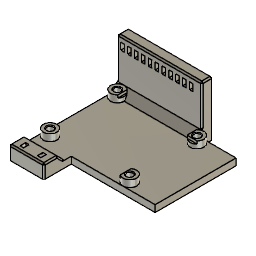
Pi Mount v3 (Autodesk Fusion 360 design; units mm, degrees)
Autodesk Fusion 360 part; units mm, degrees
note: some values were not read from the file. Set by a fixed rule: which sketch regions a step uses.
sketch "Sketch1" plane through (0, 0, 0) normal (0, 0, 1) x (1, 0, 0)
  line L0 (0, 0) -> (85, 0) construction
  line L1 (85, 0) -> (85, 56) construction
  line L2 (85, 56) -> (0, 56) construction
  line L3 (0, 56) -> (0, 0) construction
  line L4 (61.5, 3.5) -> (3.5, 3.5) construction
  line L5 (3.5, 3.5) -> (3.5, 52.5) construction
  line L6 (3.5, 52.5) -> (61.5, 52.5) construction
  line L7 (61.5, 52.5) -> (61.5, 3.5) construction
  line L8 (61.5, 3.5) -> (3.5, 52.5) construction
  line L9 (3.5, 3.5) -> (61.5, 52.5) construction
  circle A0 centre (3.5, 52.5) radius 5
  circle A1 centre (61.5, 52.5) radius 5
  circle A2 centre (61.5, 3.5) radius 5
  circle A3 centre (3.5, 3.5) radius 5
  point P0 (32.5, 28)
  dimension "d1" = 85
  dimension "d2" = 56
  dimension "d3" = 3.5
  dimension "d4" = 3.5
  dimension "d5" = 3.5
  dimension "d6" = 58
  dimension "d7" = 10
  constraint horizontal L0
  constraint vertical L1
  constraint horizontal L2
  constraint vertical L3
  constraint coincident L0.start L3.end
  constraint horizontal L4
  constraint perpendicular L4 L5
  constraint parallel L4 L6
  constraint parallel L5 L7
  constraint coincident L8 P0
  constraint coincident L9 P0
  constraint coincident L5.end L6.start
  constraint coincident L6.end L7.start
  constraint coincident L4.start L7.end
  constraint coincident L4.end L5.start
  constraint equal A2 A3
  constraint equal A1 A2
  constraint equal A0 A1
  measures "d1" distance of L0.start L0.end
  measures "d2" distance of L0.start L2.end
  measures "d3" distance of L2 L6
  measures "d4" distance of L3 L5
  measures "d5" distance of L0 L4
  measures "d6" distance of L5.end L6.end
  measures "d7" diameter of A0
extrude "Extrude1" add sketch "Sketch1" against normal blind 5 makes body 1 at (66.4938, 52.2508, -3.3333) makes body 2 at (66.4938, 3.2508, -3.3333) makes body 3 at (8.4938, 52.2508, -3.3333) makes body 4 at (8.4938, 3.2508, -3.3333)
sketch "Sketch2" plane through (0, 0, -5) normal (0, 0, -1) x (1, 0, 0)
  circle A0 centre (3.5, -3.5) radius 5
  circle A1 centre (61.5, -3.5) radius 5
  circle A2 centre (61.5, -52.5) radius 5
  circle A3 centre (3.5, -52.5) radius 5
  line L0 (-1.5, 1.5) -> (85, 1.5)
  line L1 (85, 1.5) -> (85, -57.5)
  line L2 (85, -57.5) -> (-1.5, -57.5)
  line L3 (-1.5, -57.5) -> (-1.5, 1.5)
  line L4 (85, 0) -> (85, -56)
  circle A4 centre (3.5, -3.5) radius 5
  circle A5 centre (3.5, -52.5) radius 5
  constraint horizontal L0
  constraint vertical L1
  constraint horizontal L2
  constraint vertical L3
  constraint collinear L1 L4
  constraint tangent L3 A4
  constraint tangent L0 A4
  constraint tangent L2 A5
extrude "Extrude2" add sketch "Sketch2" along normal blind 5 contours A0 A4 | A2 | A1 | A0 A3 L0 L1 L2 L3 L4 A4 A5 | A0 L0 L3 A4 | A3 A5 | A3 L2 L3 A5 bodies 1 2 3 4
sketch "Sketch4" plane through (0, 0, -10) normal (0, 0, -1) x (1, 0, 0)
  line L0 (85, -57.5) -> (85, 1.5)
  line L1 (85, 1.5) -> (-1.5, 1.5)
  line L2 (-1.5, 1.5) -> (-1.5, -57.5)
  line L3 (-1.5, -57.5) -> (85, -57.5)
  line L4 (-1.5, -57.5) -> (60, -57.5)
  line L5 (60, -57.5) -> (60, -65.5)
  line L6 (60, -65.5) -> (-1.5, -65.5)
  line L7 (-1.5, -65.5) -> (-1.5, -57.5)
  dimension "d17" = 61.5
  dimension "d18" = 8
  constraint horizontal L4
  constraint vertical L5
  constraint horizontal L6
  constraint vertical L7
  constraint coincident L2.end L3.start
  measures "d17" distance of L2.end L4.end
  measures "d18" distance of L2.end L6.end
extrude "Extrude3" add sketch "Sketch4" against normal blind 40 contours L3 L4 L5 L6 L7 bodies 1
ref_plane "WorkPlane1" through (29.25, 61.5, 26) normal (0, 0, 1) x (1, 0, 0)
sketch "Sketch5" plane through (0, 0, 26) normal (0, 0, 1) x (1, 0, 0)
  line L0 (60, 65.5) -> (-1.5, 65.5)
  line L1 (-1.5, 65.5) -> (-1.5, 57.5)
  line L2 (-1.5, 57.5) -> (60, 57.5)
  line L3 (60, 57.5) -> (60, 65.5)
  line L4 (1, 57.5) -> (3.5, 57.5)
  line L5 (3.5, 57.5) -> (3.5, 65.5)
  line L6 (3.5, 65.5) -> (1, 65.5)
  line L7 (1, 65.5) -> (1, 57.5)
  line L8 (8.5, 57.5) -> (8.5, 65.5)
  line L9 (6, 65.5) -> (6, 57.5)
  line L10 (8.5, 65.5) -> (6, 65.5)
  line L11 (6, 57.5) -> (8.5, 57.5)
  line L12 (13.5, 57.5) -> (13.5, 65.5)
  line L13 (11, 65.5) -> (11, 57.5)
  line L14 (13.5, 65.5) -> (11, 65.5)
  line L15 (11, 57.5) -> (13.5, 57.5)
  line L16 (18.5, 57.5) -> (18.5, 65.5)
  line L17 (16, 65.5) -> (16, 57.5)
  line L18 (18.5, 65.5) -> (16, 65.5)
  line L19 (16, 57.5) -> (18.5, 57.5)
  line L20 (23.5, 57.5) -> (23.5, 65.5)
  line L21 (21, 65.5) -> (21, 57.5)
  line L22 (23.5, 65.5) -> (21, 65.5)
  line L23 (21, 57.5) -> (23.5, 57.5)
  line L24 (28.5, 57.5) -> (28.5, 65.5)
  line L25 (26, 65.5) -> (26, 57.5)
  line L26 (28.5, 65.5) -> (26, 65.5)
  line L27 (26, 57.5) -> (28.5, 57.5)
  line L28 (33.5, 57.5) -> (33.5, 65.5)
  line L29 (31, 65.5) -> (31, 57.5)
  line L30 (33.5, 65.5) -> (31, 65.5)
  line L31 (31, 57.5) -> (33.5, 57.5)
  line L32 (38.5, 57.5) -> (38.5, 65.5)
  line L33 (36, 65.5) -> (36, 57.5)
  line L34 (38.5, 65.5) -> (36, 65.5)
  line L35 (36, 57.5) -> (38.5, 57.5)
  line L36 (43.5, 57.5) -> (43.5, 65.5)
  line L37 (41, 65.5) -> (41, 57.5)
  line L38 (43.5, 65.5) -> (41, 65.5)
  line L39 (41, 57.5) -> (43.5, 57.5)
  line L40 (48.5, 57.5) -> (48.5, 65.5)
  line L41 (46, 65.5) -> (46, 57.5)
  line L42 (48.5, 65.5) -> (46, 65.5)
  line L43 (46, 57.5) -> (48.5, 57.5)
  line L44 (53.5, 57.5) -> (53.5, 65.5)
  line L45 (51, 65.5) -> (51, 57.5)
  line L46 (53.5, 65.5) -> (51, 65.5)
  line L47 (51, 57.5) -> (53.5, 57.5)
  dimension "d22" = 2.5
  dimension "d23" = 2.5
  dimension "d26" = 5
  dimension "d27" = 0
  constraint horizontal L4
  constraint vertical L5
  constraint horizontal L6
  constraint vertical L7
  constraint coincident L0 L5.end
  constraint coincident L2 L4.start
  measures "d22" distance of L4.start L4.end
  measures "d23" distance of L1 L7
extrude "Extrude4" cut sketch "Sketch5" against normal blind 5 contours L0 L2 L44 L45 L46 L47 | L0 L2 L40 L41 L42 L43 | L0 L2 L36 L37 L38 L39 | L0 L2 L32 L33 L34 L35 | L0 L2 L28 L29 L30 L31 | L0 L2 L24 L25 L26 L27 | L0 L2 L20 L21 L22 L23 | L0 L2 L16 L17 L18 L19 | L0 L2 L12 L13 L14 L15 | L0 L2 L8 L9 L10 L11 | L0 L2 L4 L5 L6 L7 bodies 1
fillet "Fillet1" radius 1.25 20 edges at (3.5, 65.5, 23.5) (6, 65.5, 23.5) (8.5, 65.5, 23.5) (11, 65.5, 23.5) (13.5, 65.5, 23.5) (16, 65.5, 23.5) (18.5, 65.5, 23.5) (21, 65.5, 23.5) (23.5, 65.5, 23.5) (26, 65.5, 23.5) (28.5, 65.5, 23.5) (31, 65.5, 23.5) (33.5, 65.5, 23.5) (36, 65.5, 23.5) (38.5, 65.5, 23.5) (41, 65.5, 23.5) (43.5, 65.5, 23.5) (46, 65.5, 23.5) (48.5, 65.5, 23.5) (51, 65.5, 23.5) on bodies 1
sketch "Sketch6" plane through (0, 0, -10) normal (0, 0, -1) x (1, 0, 0)
  line L0 (60, -65.5) -> (60, -57.5)
  line L1 (60, -57.5) -> (85, -57.5)
  line L2 (85, -57.5) -> (85, 1.5)
  line L3 (85, 1.5) -> (-1.5, 1.5)
  line L4 (-1.5, 1.5) -> (-1.5, -65.5)
  line L5 (-1.5, -65.5) -> (60, -65.5)
  line L6 (-1.5, 1.5) -> (23.9, 1.5)
  line L7 (23.9, 1.5) -> (23.9, 21.5)
  line L8 (23.9, 21.5) -> (-1.5, 21.5)
  line L9 (-1.5, 21.5) -> (-1.5, 1.5)
  line L10 (11.2, 21.5) -> (11.2, 1.5) construction
  circle A0 centre (3.5, -3.5) radius 5 construction
  dimension "d33" = 7.7
  dimension "d34" = 12.7
  dimension "d35" = 12.7
  dimension "d36" = 20
  constraint horizontal L6
  constraint vertical L7
  constraint horizontal L8
  constraint vertical L9
  constraint coincident L3.end L4.start
  constraint coincident L8 L10.start
  constraint coincident L6 L10.end
  constraint perpendicular L6 L10
  measures "d33" distance of L10 A0.centre
  measures "d34" distance of L9 L10
  measures "d35" distance of L7 L10
  measures "d36" distance of L6.end L7.end
extrude "Extrude5" add sketch "Sketch6" against normal blind 5 contours L3 L6 L7 L8 L9 bodies 1
sketch "Sketch7" plane through (0, -21.5, 0) normal (0, -1, 0) x (1, 0, 0)
  line L0 (-1.5, -10) -> (23.9, -10)
  line L1 (23.9, -10) -> (23.9, -5)
  line L2 (23.9, -5) -> (-1.5, -5)
  line L3 (-1.5, -5) -> (-1.5, -10)
  line L4 (23.9, -5) -> (-1.5, -5)
  line L5 (-1.5, -5) -> (-1.5, 0)
  line L6 (-1.5, 0) -> (23.9, 0)
  line L7 (23.9, 0) -> (23.9, -5)
  dimension "d39" = 5
  constraint horizontal L4
  constraint vertical L5
  constraint horizontal L6
  constraint vertical L7
  constraint coincident L1.end L2.start
  constraint collinear L3 L5
  measures "d39" distance of L2.end L5.end
extrude "Extrude6" add sketch "Sketch7" against normal blind 10 contours L2 L4 L5 L6 L7 bodies 1
ref_plane "WorkPlane2" through (11.2, -16.5, -5) normal (0, -1, 0) x (1, 0, 0)
sketch "Sketch8" plane through (0, -16.5, 0) normal (0, -1, 0) x (-1, 0, 0)
  line L0 (1.5, 0) -> (-23.9, 0)
  line L1 (-23.9, 0) -> (1.5, 0)
  ellipse E0 centre (-11.2, 0) end of major axis (-18.7, 0) minor radius 5
  line L2 (-3.7, 0) -> (-18.7, 0) construction
  line L3 (-11.2, 5) -> (-11.2, -5) construction
  spline S0 degree 3 poles (-6.2, 0) (-6.2, 0.2136) (-6.2636, 0.4716) (-6.5744, 0.8398) (-6.9638, 1.3009) (-7.7837, 1.8539) (-8.8758, 2.1755) (-10.1221, 2.5425) (-11.6823, 2.5974) (-13.0027, 2.3088) (-14.1231, 2.0639) (-15.0493, 1.5776) (-15.5677, 1.1057) (-16.0026, 0.7099) (-16.1498, 0.3716) (-16.1882, 0.1411) (-16.226, -0.086) (-16.2065, -0.2804) (-15.9927, -0.6144) (-15.7383, -1.012) (-15.1288, -1.5532) (-14.2014, -1.9373) (-13.0663, -2.4075) (-11.5022, -2.6125) (-10.0863, -2.4284) (-8.7831, -2.2589) (-7.6344, -1.7622) (-6.9839, -1.2357) (-6.4805, -0.8283) (-6.2827, -0.4507) (-6.2242, -0.2025) (-6.2071, -0.13) (-6.2, -0.0649) (-6.2, 0) knots -3.141593 -3.141593 -3.141593 -3.141593 -2.628909 -2.628909 -2.628909 -1.986734 -1.986734 -1.986734 -1.253989 -1.253989 -1.253989 -0.632204 -0.632204 -0.632204 -0.110599 -0.110599 -0.110599 0.40321 0.40321 0.40321 1.014846 1.014846 1.014846 1.763467 1.763467 1.763467 2.45253 2.45253 2.45253 2.985813 2.985813 2.985813 3.141593 3.141593 3.141593 3.141593
  dimension "d42" = 15
  dimension "d43" = 10
  dimension "d55" = -2.5
  constraint coincident E0 L2.start
  constraint coincident E0 L2.end
  constraint coincident E0 L3.start
  constraint coincident E0 L3.end
  constraint midpoint L0 E0.centre
  constraint parallel L0 L2
  measures "d42" distance of E0
extrude "Extrude10" cut sketch "Sketch8" along normal mid plane 4 contours L0 L1 E0 S0 | L0 L1 E0 S0 bodies 1
chamfer "Chamfer2" distance 5 angle 45 1 edges at (11.2, -11.5, -5) on bodies 1
sketch "Sketch9" plane through (-1.5, 0, 0) normal (-1, 0, 0) x (0, -1, 0)
  line L0 (-52.5, -5) -> (-57.5, -5)
  line L1 (-57.5, -5) -> (-57.5, 30)
  line L2 (-57.5, 30) -> (-65.5, 30)
  line L3 (-65.5, 30) -> (-65.5, -10)
  line L4 (-65.5, -10) -> (21.5, -10)
  line L5 (21.5, -10) -> (21.5, 0)
  line L6 (21.5, 0) -> (11.5, 0)
  line L7 (6.5, -5) -> (-3.5, -5)
  line L8 (-3.5, -5) -> (-52.5, -5)
  line L9 (-57.5, 0) -> (-52.5, -5)
  line L10 (11.5, 0) -> (6.5, -5)
  dimension "d51" = 45
  dimension "d52" = 5
  constraint coincident L1 L9.start
  constraint coincident L0 L8.end
  measures "d51" angle of L0 L9
  measures "d52" distance of L0 L9.start
extrude "Extrude9" add sketch "Sketch9" against normal up to surface (61.5 mm away) contours L0 L1 L9 bodies 1
sketch "Sketch3" plane through (0, 0, 0) normal (0, 0, 1) x (-1, 0, 0)
  circle A0 centre (-3.5, -52.5) radius 5
  circle A1 centre (-3.5, -3.5) radius 5
  circle A2 centre (-61.5, -3.5) radius 5
  circle A3 centre (-61.5, -52.5) radius 5
hole "Hole1" at (3.5, 52.5, 0) at (61.5, 52.5, 0) at (61.5, 3.5, 0) at (3.5, 3.5, 0) direction (0, 0, -1) diameter 4.6 depth 6 tip angle 118 countersink diameter 5.6 countersink angle 90 bodies 1
chamfer "Chamfer1" distance 1 angle 45 15 edges at (-1.5, 61.5, 30) (-1.5, 65.5, 10) (-1.5, 57.5, 15) (29.25, 57.5, 30) (29.25, 65.5, 30) (60, 61.5, 30) (60, 65.5, 10) (60, 57.5, 15) (-1.5, -16.5, 0) (-1.5, -9, -2.5) (-1.5, -21.5, -5) (11.2, -21.5, 0) (23.9, -16.5, 0) (23.9, -21.5, -5) (23.9, -9, -2.5) on bodies 1
sketch "Sketch10" plane through (0, 0, 0) normal (0, 0, 1) x (-1, 0, 0)
  circle A0 centre (-3.5, -52.5) radius 2.8
  circle A1 centre (-3.5, -52.5) radius 5
  circle A2 centre (-61.5, -3.5) radius 2.8
  circle A3 centre (-61.5, -3.5) radius 5
  circle A4 centre (-61.5, -52.5) radius 2.8
  circle A5 centre (-61.5, -52.5) radius 5
  circle A6 centre (-3.5, -3.5) radius 2.8
  circle A7 centre (-3.5, -3.5) radius 5
  line L0 (-7.2, -49.137) -> (-7.2, -55.863)
  line L1 (-57.8, -55.863) -> (-57.8, -49.137)
  line L2 (-65.0707, -49) -> (-57.9293, -49)
  line L3 (-58.5, -7.5) -> (-58.5, 0.5)
  dimension "d58" = 3.7
  dimension "d59" = 3.7
  dimension "d60" = 3.5
  dimension "d61" = 3
  constraint coincident A1 L0.start
  constraint coincident A1 L0.end
  constraint vertical L0
  constraint coincident A5 L1.start
  constraint coincident A5 L1.end
  constraint vertical L1
  constraint coincident A5 L2.start
  constraint coincident A5 L2.end
  constraint horizontal L2
  constraint coincident A3 L3.start
  constraint coincident A3 L3.end
  constraint vertical L3
  measures "d58" distance of A0.centre L0
  measures "d59" distance of A4.centre L1
  measures "d60" distance of A4.centre L2
  measures "d61" distance of A2.centre L3
extrude "Extrude11" cut sketch "Sketch10" against normal blind 2 contours A1 L0 | A3 L3 | A5 L1 | A5 L2 picked at (-7.3514, -51.5725) picked at (-57.5568, -3.0636) bodies 1
equation "d17 = 58 mm + 3.5 mm"
equation "d31 = ( 2.5 / 2 ) * 1 mm"
equation "d35 = d34"
